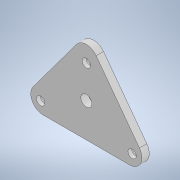
# Autodesk Inventor part: Idle Ball Mount
Saved by Autodesk Inventor 2022 (Build 260153000, 153)
## iProperties
Created: 2022-08-27
Part Number: Idle Ball Mount
Material: Generic
Document SubType Name: Modeling
Designer: Nick
Density: 1 g/cm^3
Appearance: Default
Author: Nick
Autodesk Inventor part; units mm, degrees
ref_plane "YZ Plane" through (0, 0, 0) normal (1, 0, 0) x (0, 1, 0)
ref_plane "XZ Plane" through (0, 0, 0) normal (0, 1, 0) x (-1, 0, 0)
ref_plane "XY Plane" through (0, 0, 0) normal (0, 0, 1) x (1, 0, 0)
sketch "Sketch1" plane through (0, 0, 0) normal (0, 0, 1) x (1, 0, 0)
  line L0 (18.6512, 0) -> (-18.6512, 0) construction
  line L1 (-27.5858, -4.4915) -> (0, 32.6237)
  line L2 (0, 32.6237) -> (27.5858, -4.4915)
  line L3 (27.5858, -4.4915) -> (-27.5858, -4.4915)
  line L4 (0, 32.6237) -> (0, 9.3762) construction
  line L5 (0, 9.3762) -> (-27.5858, -4.4915) construction
  line L6 (0, 9.3762) -> (27.5858, -4.4915) construction
  point P0 (0, 0)
  point P1 (0, 22.6237)
  point P2 (0, 0)
  dimension "d0" = 37.3025
  dimension "d1" = 22.6237
  dimension "d2" = 10
  dimension "d3" = 10
  dimension "d21" = 26.689
  dimension "d22" = 26.689
  constraints: 14 end point, 3 point on line, 3 vertical alignment, 2 coincident, 2 horizontal, 1 equal length, 1 horizontal alignment, 1 midpoint, 1 vertical
  measures "d0" distance of L0.start L0.end
  measures "d1" distance from line of point (0, 22.624) L0
  measures "d2" distance of L1.end point (0, 22.624)
  measures "d3" distance of L1.start L0.end
  measures "d21" angle of L2 L6
  measures "d22" angle of L3 L6
extrude "Extrusion1" add sketch "Sketch1" along normal blind 3
hole "Hole1" at (0, 22.6237, 0) at (18.6512, 0, 0) at (-18.6512, 0, 0) direction (0, 0, 1) diameter 3.4 depth 7 tip angle 118 countersink diameter 6.3 countersink angle 90 clearance for "Flat Head Machine Screw" size "M3" standard "Ansi Metric M Profile"
hole "Hole2" at (0, 9.3762, 0) direction (0, 0, 1) diameter 4.5 depth 7 tip angle 118 clearance for "Flat Head Machine Screw" size "M4" standard "Ansi Metric M Profile"
fillet "Fillet1" radius 5 3 edges at (0, 32.6237, 1.5) (27.5858, -4.4915, 1.5) (-27.5858, -4.4915, 1.5)
equation "\"d21\" = d22"
body "Solid1"
